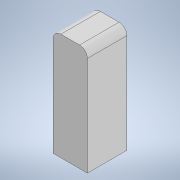
# Autodesk Inventor part: 10000 mAh battery
Saved by Autodesk Inventor 2020 (Build 240168000, 168)
## iProperties
Created: 2019-09-18
Part Number: 10000 mAh battery
Material: Generic
Document SubType Name: Modeling
Designer: User
Density: 1 g/cm^3
Appearance: Default
Author: User
Autodesk Inventor part; units mm, degrees
ref_plane "YZ Plane" through (0, 0, 0) normal (1, 0, 0) x (0, 1, 0)
ref_plane "XZ Plane" through (0, 0, 0) normal (0, 1, 0) x (-1, 0, 0)
ref_plane "XY Plane" through (0, 0, 0) normal (0, 0, 1) x (1, 0, 0)
sketch "Sketch1" plane through (0, 0, 0) normal (0, 1, 0) x (-1, 0, 0)
  line L0 (-27.9337, 32.1945) -> (27.9336, 32.1945)
  line L1 (27.9336, 32.1945) -> (27.9337, -32.1945)
  line L2 (27.9337, -32.1945) -> (-27.9336, -32.1945)
  line L3 (-27.9336, -32.1945) -> (-27.9337, 32.1945)
  line L4 (-27.9337, 32.1945) -> (27.9337, -32.1945) construction
  line L5 (27.9336, 32.1945) -> (-27.9336, -32.1945) construction
  point P0 (0, 0)
  dimension "d0" = 64.389
  dimension "d1" = 55.8673
  constraints: 12 end point, 2 midpoint, 2 parallel, 1 horizontal, 1 perpendicular
  measures "d0" distance of L0.end L1.end
  measures "d1" distance of L0.start L0.end
extrude "Extrusion1" add sketch "Sketch1" along normal blind 174.625
fillet "Fillet1" radius 12.7 2 edges at (-27.9337, 174.625, 0) (27.9337, 174.625, 0)
body "Solid1"
